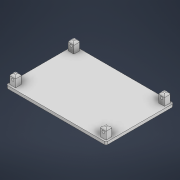
# Autodesk Inventor part: RPIholderTOP
Saved by Autodesk Inventor 2022 (Build 260153000, 153)
## iProperties
Created: 2023-11-26
Part Number: RPIholderTOP
Material: Všeobecné
Document SubType Name: Modeling
Designer: tada
Density: 1 g/cm^3
Appearance: Výchozí
Author: tada
Autodesk Inventor part; units mm, degrees
ref_plane "YZ Plane" through (0, 0, 0) normal (1, 0, 0) x (0, 1, 0)
ref_plane "XZ Plane" through (0, 0, 0) normal (0, 1, 0) x (-1, 0, 0)
ref_plane "XY Plane" through (0, 0, 0) normal (0, 0, 1) x (1, 0, 0)
sketch "Náčrt1" plane through (0, 0, 0) normal (0, 1, 0) x (-1, 0, 0)
  line L0 (0, 0) -> (-106, 0)
  line L1 (-106, 0) -> (-106, -72)
  line L2 (-106, -72) -> (0, -72)
  line L3 (0, -72) -> (0, 0)
  dimension "d0" = 106
  dimension "d1" = 72
  constraints: 8 end point, 2 parallel, 1 horizontal, 1 perpendicular
  measures "d0" distance of L1.end L2.end
  measures "d1" distance between parallel lines of L0 L2
extrude "Vysunutí1" add sketch "Náčrt1" along normal blind 3
sketch "Náčrt2" plane through (0, 3, 0) normal (0, 1, 0) x (1, 0, 0)
  line L0 (0, 72) -> (0, 0) projected
  line L1 (106, 0) -> (106, 72) projected
  line L2 (0, 0) -> (106, 0)
  line L3 (106, 0) -> (106, 72)
  line L4 (106, 72) -> (0, 72)
  line L5 (0, 72) -> (0, 0)
  line L6 (2, 70) -> (104, 70)
  line L7 (104, 70) -> (104, 2)
  line L8 (104, 2) -> (2, 2)
  line L9 (2, 2) -> (2, 70)
  line L10 (2, 2) -> (8, 2)
  line L11 (8, 2) -> (8, 8)
  line L12 (8, 8) -> (2, 8)
  line L13 (2, 8) -> (2, 2)
  line L14 (2, 70) -> (8, 70)
  line L15 (8, 70) -> (8, 64)
  line L16 (8, 64) -> (2, 64)
  line L17 (2, 64) -> (2, 70)
  line L18 (53, -6.8672) -> (53, 83.3894) construction
  line L19 (104, 2) -> (104, 70)
  line L20 (104, 2) -> (98, 2)
  line L21 (98, 2) -> (98, 8)
  line L22 (98, 8) -> (104, 8)
  line L23 (104, 8) -> (104, 2)
  line L24 (104, 70) -> (98, 70)
  line L25 (98, 70) -> (98, 64)
  line L26 (98, 64) -> (104, 64)
  line L27 (104, 64) -> (104, 70)
  point P0 (2, 64)
  dimension "d4" = 2
  dimension "d5" = 6
  dimension "d6" = 6
  dimension "d7" = 6
  dimension "d8" = 6
  constraints: 52 end point, 8 parallel, 6 symmetric about line, 4 perpendicular, 3 horizontal, 2 vertical, 3 other
  measures "d4" distance between parallel lines of L4 L6
  measures "d5" distance between parallel lines of L13 L11
  measures "d6" distance between parallel lines of L10 L12
  measures "d7" distance between parallel lines of L14 L16
  measures "d8" distance between parallel lines of L17 L15
extrude "Vysunutí2" add sketch "Náčrt2" along normal blind 10 contours L6 L15 L16 L9 | L6 L7 L26 L25 | L12 L11 L8 L9 | L7 L8 L21 L22
sketch "Náčrt3" plane through (2, 3, -2) normal (0, 0, 1) x (1, 0, 0)
  circle A0 centre (3, 6) radius 1.3
  line L0 (0, 10) -> (6, 10) projected
  line L1 (6, 0) -> (6, 10) projected
  line L2 (-2, 0) -> (104, 0) projected
  circle A1 centre (99, 6) radius 1.3
  line L3 (96, 10) -> (102, 10) projected
  line L4 (102, 0) -> (102, 10) projected
  point P0 (-2, -3)
  dimension "d11" = 2.6
  dimension "d12" = 4
  dimension "d13" = 3
  dimension "d14" = 6
  dimension "d15" = 2.6
  dimension "d16" = 4
  dimension "d17" = 3
  dimension "d18" = 6
  constraints: 2 centre point
  measures "d11" diameter of A0
  measures "d12" distance from line of L0 A0.centre
  measures "d13" distance from line of L1 A0.centre
  measures "d14" distance from line of A0.centre L2
  measures "d15" diameter of A1
  measures "d16" distance from line of L3 A1.centre
  measures "d17" distance from line of L4 A1.centre
  measures "d18" distance from line of L2 A1.centre
extrude "Vysunutí3" cut sketch "Náčrt3" against normal blind 100
fillet "Zaoblení1" radius 2 20 edges at (106, 1.5, 0) (106, 1.5, -72) (0, 1.5, 0) (0, 1.5, -72) (2, 13, -67) (5, 13, -70) (8, 13, -67) (5, 13, -64) (8, 13, -5) (5, 13, -8) (2, 13, -5) (5, 13, -2) (98, 13, -5) (101, 13, -2) (104, 13, -5) (101, 13, -8) (104, 13, -67) (101, 13, -70) (98, 13, -67) (101, 13, -64)
equation "\"d6\" = d5"
equation "\"d7\" = d5"
equation "\"d8\" = d5"
